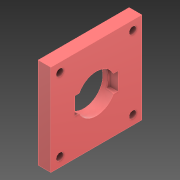
# Autodesk Inventor part: conischLagerBlok
Saved by Autodesk Inventor 2020 (Build 240168000, 168)
## iProperties
Created: 2020-05-25
Part Number: conischLagerBlok
Material: Generic
Document SubType Name: Modeling
Designer: stefa
Density: 1 g/cm^3
Appearance: Smooth - Red
Author: stefa
Autodesk Inventor part; units mm, degrees
ref_plane "YZ Plane" through (0, 0, 0) normal (1, 0, 0) x (0, 1, 0)
ref_plane "XZ Plane" through (0, 0, 0) normal (0, 1, 0) x (-1, 0, 0)
ref_plane "XY Plane" through (0, 0, 0) normal (0, 0, 1) x (1, 0, 0)
sketch "Sketch1" plane through (0, 0, 0) normal (0, 1, 0) x (-1, 0, 0)
  line L0 (23.3994, 10.5) -> (23.3994, -10.5) projected
  arc A0 (30.3994, 10.5) -> (23.3994, 10.5) centre (26.8994, -1.5) ccw
  line L1 (30.3994, 10.5) -> (30.3994, -10.5) projected
  arc A1 (23.3994, -10.5) -> (30.3994, -10.5) centre (26.8994, 1.5) ccw
  line L2 (30.3994, 0) -> (23.3994, 0)
  line L3 (30.3994, -10.5) -> (30.3994, -25)
  line L4 (30.3994, -25) -> (23.3994, -25)
  line L5 (23.3994, -25) -> (23.3994, -10.5)
  line L6 (30.3994, 10.5) -> (30.3994, 25)
  line L7 (30.3994, 25) -> (23.3994, 25)
  line L8 (23.3994, 25) -> (23.3994, 10.5)
  arc A2 (23.3994, -10.6041) -> (30.3994, -10.6041) centre (26.8994, 1.5) ccw
  arc A3 (30.3994, 10.6041) -> (23.3994, 10.6041) centre (26.8994, -1.5) ccw
  point P0 (0, 0)
  dimension "d0" = 25
  dimension "d1" = 25
  dimension "d22" = 0.1
  dimension "d23" = 0.1
  constraints: 14 end point, 8 point on circle, 4 centre point, 4 point on line, 3 perpendicular, 2 midpoint, 2 vertical, 1 parallel, 5 other
  measures "d0" distance between parallel lines of L2 L4
  measures "d1" distance between parallel lines of L7 L2
  measures "d22" radial gap between concentric circles of A1 A2
  measures "d23" radial gap between concentric circles of A0 A3
revolve "Revolution1" add sketch "Sketch1" angle 360 about axis through (-30.3994, 0, 0) along (1, 0, 0) contours L8 L7 L6 A3
sketch "Sketch2" plane through (-23.3994, 0, 0) normal (1, 0, 0) x (0, 0, -1)
  circle A0 centre (0, 0) radius 25 projected
  line L0 (-11.9, 4.9) -> (11.9, 4.9)
  line L1 (11.9, 4.9) -> (11.9, -4.9)
  line L2 (11.9, -4.9) -> (-11.9, -4.9)
  line L3 (-11.9, -4.9) -> (-11.9, 4.9)
  line L4 (-11.9, 4.9) -> (11.9, -4.9) construction
  line L5 (11.9, 4.9) -> (-11.9, -4.9) construction
  point P0 (0, 0)
  dimension "d3" = 23.8
  dimension "d4" = 9.8
  constraints: 12 end point, 2 midpoint, 2 parallel, 1 horizontal, 1 perpendicular
  measures "d3" distance of L1.end L2.end
  measures "d4" distance of L0.end L1.end
extrude "Extrusion1" cut sketch "Sketch2" against normal blind 4.5 contours L0 L1 L2 L3
sketch "Sketch3" plane through (-23.3994, 0, 0) normal (1, 0, 0) x (0, 0, -1)
  circle A0 centre (0, 0) radius 25 projected
  line L0 (11.9, -4.9) -> (9.4041, -4.9) projected
  line L1 (-11.9, -4.9) -> (-11.9, 4.9) projected
  line L2 (-11.9, 4.9) -> (-9.4041, 4.9) projected
  line L3 (9.4041, 4.9) -> (11.9, 4.9) projected
  line L4 (11.9, 4.9) -> (11.9, -4.9) projected
  line L5 (-9.4041, -4.9) -> (-11.9, -4.9) projected
  circle A1 centre (0, 0) radius 20
  line L6 (-25, 25) -> (25, 25)
  line L7 (25, 25) -> (25, -25)
  line L8 (25, -25) -> (-25, -25)
  line L9 (-25, -25) -> (-25, 25)
  line L10 (-25, 25) -> (25, -25) construction
  line L11 (25, 25) -> (-25, -25) construction
  circle A2 centre (20, -20) radius 2
  circle A3 centre (20, 20) radius 2
  circle A4 centre (-20, -20) radius 2
  circle A5 centre (-20, 20) radius 2
  arc A6 (-9.4041, -4.9) -> (9.4041, -4.9) centre (0, 0) ccw projected
  arc A7 (9.4041, 4.9) -> (-9.4041, 4.9) centre (0, 0) ccw projected
  point P0 (0, 0)
  point P1 (-25, 0)
  point P2 (0, -25)
  point P3 (0, 25)
  point P4 (25, 0)
  dimension "d7" = 40
  dimension "d8" = 50
  dimension "d9" = 50
  dimension "d12" = 4
  dimension "d13" = 5
  dimension "d16" = 40
  dimension "d19" = 40
  constraints: 12 end point, 5 centre point, 2 horizontal, 2 midpoint, 2 parallel, 1 perpendicular, 1 point on line, 1 vertical, 6 other
  measures "d7" diameter of A1
  measures "d8" distance of L7.end L8.end
  measures "d9" distance of L6.end L7.end
  measures "d12" diameter of A2
  measures "d13" distance from line of L8 A2.centre
  measures "d16" distance of A2.centre A3.centre
  measures "d19" distance of A2.centre A4.centre
extrude "Extrusion2" add sketch "Sketch3" against normal up to surface (7 mm away) contours A0 | L7 L8 A0 | A0 L6 L7 | A0 L9 L6 | L8 L9 A0
equation "\"d1\" = d0"
equation "\"d16\" = d8 - 2 * d13"
equation "\"d19\" = d8 - 2 * d13"
body "Solid1"
